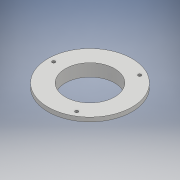
# Autodesk Inventor part: ACO.RODA25-02
Saved by Autodesk Inventor 2018 (Build 220112000, 112)
## iProperties
Created: 2018-02-28
Part Number: ACO.RODA25-02
Material: Generic
Document SubType Name: Modeling
Designer: isai
Density: 1 g/cm^3
Appearance: Default
Author: isai
Autodesk Inventor part; units mm, degrees
ref_plane "YZ Plane" through (0, 0, 0) normal (1, 0, 0) x (0, 1, 0)
ref_plane "XZ Plane" through (0, 0, 0) normal (0, 1, 0) x (-1, 0, 0)
ref_plane "XY Plane" through (0, 0, 0) normal (0, 0, 1) x (1, 0, 0)
sketch "Sketch1" plane through (0, 0, 0) normal (0, 0, 1) x (1, 0, 0)
  circle A0 centre (0, 0) radius 23.75
  circle A1 centre (0, 0) radius 25.5
  circle A2 centre (0, 0) radius 40.5
  dimension "d0" = 47.5
  dimension "d15" = 81
  dimension "d17" = 51
  constraints: 3 centre point, 1 coincident
  measures "d0" diameter of A0
  measures "d15" diameter of A2
  measures "d17" diameter of A1
extrude "Extrusion1" add sketch "Sketch1" against normal blind 4 contours A2
extrude "Extrusion2" add sketch "Sketch1" against normal blind 12 contours A1
sketch "Sketch2" plane through (0, 0, -4) normal (0, 0, -1) x (-1, 0, 0)
  circle A0 centre (0, 0) radius 25.5 projected
  circle A1 centre (0, 0) radius 40.5 projected
  circle A2 centre (35, 0) radius 1.5
  circle A3 centre (-17.5, 30.3109) radius 1.5
  circle A4 centre (-17.5, -30.3109) radius 1.5
  dimension "d7" = 3
  dimension "d8" = 35
  dimension "d11" = 360
  constraints: 3 centre point, 7 other
  measures "d7" diameter of A2
  measures "d8" distance of point (0, 0) A2.centre
extrude "Extrusion3" cut sketch "Sketch2" against normal blind 12 contours A2 | A3 | A4
equation "\"d0\" = a"
equation "\"a\" = 47.5"
body "Solid1"
